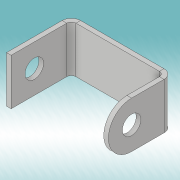
# Autodesk Inventor part: SHEET_METAL2
Saved by Autodesk Inventor 2019 (Build 230136000, 136)
## iProperties
Created: 2019-02-06
Part Number: SHEET_METAL2
Material: Generic
Document SubType Name: Sheet Metal
Designer: nelson.soberon
Density: 1 g/cm^3
Sheet Metal Rule: Default_mm
Appearance: Default
Author: nelson.soberon
Autodesk Inventor part; units mm, degrees
ref_plane "YZ Plane" through (0, 0, 0) normal (1, 0, 0) x (0, 1, 0)
ref_plane "XZ Plane" through (0, 0, 0) normal (0, 1, 0) x (-1, 0, 0)
ref_plane "XY Plane" through (0, 0, 0) normal (0, 0, 1) x (1, 0, 0)
sketch "Sketch1" plane through (0, 0, 0) normal (0, 0, 1) x (1, 0, 0)
  line L0 (0, 0) -> (44, 0)
  line L1 (44, 0) -> (44, -20)
  line L2 (44, -20) -> (0, -20)
  line L3 (0, -20) -> (0, 0)
  dimension "d0" = 44
  dimension "d1" = 20
  constraints: 8 end point, 2 parallel, 1 horizontal, 1 perpendicular
  measures "d0" distance of L1.end L2.end
  measures "d1" distance of L2.end L0.start
extrude "Extrusion1" add sketch "Sketch1" along normal mid plane 2
sketch "Sketch2" plane through (42, 0, -1) normal (1, 0, 0) x (0, 1, 0)
  line L0 (-20, 0) -> (0, 0)
  line L1 (0, 0) -> (0, 28)
  line L2 (0, 28) -> (-20, 28)
  line L3 (-20, 28) -> (-20, 0)
  constraints: 6 end point, 1 horizontal, 1 perpendicular, 1 vertical
edge flange "Flange1" height 28 angle 90 thickness 2 bend radius 2 thickness toward (1, 0, 0) relief tear relief width 2 relief depth 1 corner gap 2 corner form 0 edges at (44, -10, 1) (0, -10, 1) wall of the first edge with corners at (42, -20, -1) (42, 0, -1) (42, 0, 27) (42, -20, 27)
bend "Bend1"
corner "Corner1"
sketch "Sketch3" plane through (44, -20, 27) normal (1, 0, 0) x (0, 0, -1)
  line L0 (24, 0) -> (0, 0) projected
  line L1 (0, 0) -> (0, 20) projected
  line L2 (0, 0) -> (0, 20)
  line L3 (0, 20) -> (10, 20)
  line L4 (0, 20) -> (24, 20) projected
  line L5 (0, 0) -> (10, 0)
  arc A0 (10, 20) -> (10, 0) centre (10, 10) ccw
  circle A1 centre (10, 10) radius 4
  point P0 (27, 20)
  point P1 (0, 10)
  dimension "d15" = 10
  dimension "d16" = 8
  constraints: 6 end point, 3 coincident, 3 point on circle, 2 centre point, 2 point on line, 1 collinear, 1 midpoint
  measures "d15" distance of L1.end L3.end
  measures "d16" diameter of A1
extrude "Cut1" cut sketch "Sketch3" against normal blind 2
sketch "Sketch4" plane through (0, -20, 27) normal (-1, 0, 0) x (0, 0, 1)
  circle A0 centre (-10, 10) radius 4 projected
  circle A1 centre (-10, 10) radius 4
  point P0 (-27, 20)
  constraints: 1 centre point, 1 coincident, 1 concentric
extrude "Cut2" cut sketch "Sketch4" against normal blind 2
sketch "Sketch5" plane through (0, 0, -1) normal (0, 0, -1) x (-1, 0, 0)
  line L0 (-4, -20) -> (-4, 0) projected
  line L1 (-4, 0) -> (-40, 0) projected
  line L2 (-40, -20) -> (-4, -20) projected
  line L3 (-40, 0) -> (-40, -20) projected
  circle A0 centre (-22, -10) radius 4.5
  point P0 (0, 0)
  dimension "d21" = 9
  dimension "d22" = 18
  dimension "d23" = 10
  constraints: 1 centre point
  measures "d21" diameter of A0
  measures "d22" distance from line of L0 A0.centre
  measures "d23" distance from line of A0.centre L1
extrude "Extrusion2" add sketch "Sketch5" along normal blind 0.1 contours A0
equation "\"d17\" = Thickness"
equation "\"d19\" = Thickness"
equation "\"d4\" = Thickness"
equation "\"d5\" = BendReliefWidth"
equation "\"d6\" = BendReliefDepth"
equation "\"d7\" = MinimumRemnant"
equation "\"d8\" = TransitionRadius"
equation "\"d11\" = BendRadius"
equation "\"d12\" = CornerReliefSize"
equation "\"d13\" = GapSize"
equation "\"d14\" = JacobiRadiusSize"
equation "\"BendRadius\" = Thickness"
equation "\"BendReliefWidth\" = Thickness"
equation "\"BendReliefDepth\" = 0.5 * Thickness"
equation "\"CornerReliefSize\" = 4 * Thickness"
equation "\"MinimumRemnant\" = 2 * Thickness"
equation "\"TransitionRadius\" = BendRadius"
equation "\"JacobiRadiusSize\" = BendRadius"
equation "\"GapSize\" = Thickness"
equation "\"Thickness\" = 2"
body "Solid1"
